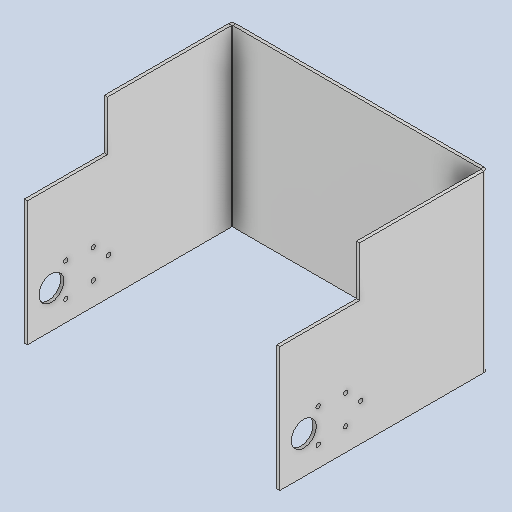
# Autodesk Inventor part: body_main_frame_new
Saved by Autodesk Inventor 2025.2 (Build 292293000, 293)
## iProperties
Created: 2025-05-30
Part Number: body_main_frame_new
Material: Aluminum 6061-AHC
Document SubType Name: Sheet Metal
Designer: chris
Density: 2.7 g/cm^3
Sheet Metal Rule: Default_mm
Appearance: Aluminum - Dark
Author: chris
Autodesk Inventor part; units mm, degrees
ref_plane "YZ Plane" through (0, 0, 0) normal (1, 0, 0) x (0, 1, 0)
ref_plane "XZ Plane" through (0, 0, 0) normal (0, 1, 0) x (-1, 0, 0)
ref_plane "XY Plane" through (0, 0, 0) normal (0, 0, 1) x (1, 0, 0)
sketch "Sketch4" plane through (0, 0, 0) normal (0, 0, 1) x (1, 0, 0)
  line L0 (-60, -42) -> (60, -42)
  line L1 (60, -42) -> (60, 42)
  line L2 (60, 42) -> (-60, 42)
  line L3 (-60, 42) -> (-60, -42)
  line L4 (-60, -42) -> (60, 42) construction
  line L5 (60, -42) -> (-60, 42) construction
  point P0 (0, 0)
  dimension "d13" = 120
  dimension "d14" = 84
  measures "d13" distance of L1.end L2.end
  measures "d14" distance of L0.end L1.end
extrude "Plate3" add sketch "Sketch4" along normal blind 1.5
sketch "Sketch5" plane through (61.5, 42, 0) normal (-1, 0, 0) x (0, -1, 0)
  line L0 (84, 0) -> (0, 0)
  line L1 (0, 0) -> (0, 100)
  line L2 (0, 100) -> (84, 100)
  line L3 (84, 100) -> (84, 0)
  line L4 (40, 5.9925) -> (78.4701, 5.9925)
  line L5 (78.4701, 5.9925) -> (78.4701, 78.464)
  line L6 (78.4701, 78.464) -> (40, 78.464)
  line L7 (40, 78.464) -> (40, 5.9925)
  constraints: 16 end point, 2 parallel, 1 horizontal, 1 perpendicular
edge flange "Flange2" height 100 angle 90 thickness 1.5 bend radius 0.31 thickness toward (-1, 0, 0) relief straight relief width 1.5 relief depth 0.75 corner gap 0.31 corner form 0 edges at (60, 0, 1.5) (-60, 0, 1.5) wall of the first edge with corners at (61.5, -42, 0) (61.5, 42, 0) (61.5, 42, 100) (61.5, -42, 100)
bend "Bend2"
corner "Corner2"
sketch "Sketch6" plane through (-61.5, -42, 100) normal (-1, 0, 0) x (0, 0, 1)
  line L0 (0, 60) -> (-38.5, 60)
  line L1 (-38.5, 60) -> (-38.5, 84)
  line L2 (-38.5, 84) -> (0, 84)
  line L3 (0, 84) -> (0, 60)
  line L4 (0, 84) -> (0, 0) projected
  line L5 (0, 0) -> (-98.19, 0) projected
  line L6 (-98.19, 84) -> (0, 84) projected
  point P0 (-100, 42)
  dimension "d26" = 38.5
  dimension "d27" = 24
  constraints: 8 end point, 2 collinear, 2 parallel, 1 horizontal, 1 perpendicular
  measures "d26" distance of L1.end L2.end
  measures "d27" distance of L2.end L0.start
extrude "Cut1" cut sketch "Sketch6" against normal blind 1.5
sketch "Sketch7" plane through (61.5, -42, 100) normal (1, 0, 0) x (0, 0, -1)
  line L0 (0, 60) -> (38.5, 60)
  line L1 (38.5, 60) -> (38.5, 84)
  line L2 (38.5, 84) -> (0, 84)
  line L3 (0, 84) -> (0, 60)
  line L4 (98.19, 0) -> (0, 0) projected
  line L5 (0, 0) -> (0, 84) projected
  line L6 (0, 84) -> (98.19, 84) projected
  point P0 (100, 42)
  dimension "d30" = 38.5
  dimension "d31" = 24
  constraints: 8 end point, 2 collinear, 2 parallel, 1 horizontal, 1 perpendicular
  measures "d30" distance of L1.end L2.end
  measures "d31" distance of L0.end L1.end
extrude "Cut2" cut sketch "Sketch7" against normal blind 1.5
sketch "Sketch8" plane through (-60, -42, 1.81) normal (1, 0, 0) x (0, 0, -1)
  point P0 (1.81, 42)
sketch "Sketch9" plane through (-60, -42, 1.81) normal (1, 0, 0) x (0, 0, -1)
  circle A0 centre (-79.79, 9.93) radius 0.7835 projected
  circle A1 centre (-66.57, 10.93) radius 0.7835 projected
  circle A2 centre (-59.27, 17.93) radius 0.7835 projected
  circle A3 centre (-79.79, 25.93) radius 0.7835 projected
  circle A4 centre (-66.57, 24.93) radius 0.7835 projected
  circle A5 centre (-86.69, 17.93) radius 6 projected
  point P0 (1.81, 42)
hole "Hole1" at (-60, -31.07, 68.38) at (-60, -24.07, 61.08) at (-60, -17.07, 68.38) at (-60, -16.07, 81.6) at (-60, -32.07, 81.6) direction (-1, 0, 0) diameter 2.1 depth 1.5
sketch "Sketch10" plane through (-60, -42, 1.81) normal (1, 0, 0) x (0, 0, -1)
  circle A0 centre (-86.69, 17.93) radius 6 projected
  point P0 (1.81, 42)
sketch "Sketch11" plane through (-60, -42, 1.81) normal (1, 0, 0) x (0, 0, -1)
  point P0 (1.81, 42)
extrude "Extrusion1" cut sketch "Sketch10" against normal blind 1.5
sketch "Sketch12" plane through (60, -42, 1.81) normal (-1, 0, 0) x (0, 0, 1)
  circle A0 centre (79.79, 25.93) radius 0.7835 projected
  circle A1 centre (79.79, 9.93) radius 0.7835 projected
  circle A2 centre (66.57, 10.93) radius 0.7835 projected
  circle A3 centre (59.27, 17.93) radius 0.7835 projected
  circle A4 centre (66.57, 24.93) radius 0.7835 projected
  point P0 (-1.81, 42)
hole "Hole2" at (60, -32.07, 81.6) at (60, -16.07, 81.6) at (60, -17.07, 68.38) at (60, -24.07, 61.08) at (60, -31.07, 68.38) direction (1, 0, 0) diameter 2.1 depth 1.5
sketch "Sketch13" plane through (60, -42, 1.81) normal (-1, 0, 0) x (0, 0, 1)
  circle A0 centre (86.69, 17.93) radius 6 projected
  point P0 (-1.81, 42)
extrude "Extrusion2" cut sketch "Sketch13" against normal blind 1.5
equation "\"d28\" = Thickness"
equation "\"d32\" = Thickness"
equation "\"d39\" = Thickness"
equation "\"d48\" = Thickness"
equation "\"d15\" = Thickness"
equation "\"d16\" = BendReliefWidth"
equation "\"d17\" = BendReliefDepth"
equation "\"d18\" = MinimumRemnant"
equation "\"d19\" = TransitionRadius"
equation "\"d22\" = BendRadius"
equation "\"d23\" = CornerReliefSize"
equation "\"d24\" = GapSize"
equation "\"d25\" = JacobiRadiusSize"
equation "\"BendReliefWidth\" = Thickness"
equation "\"BendReliefDepth\" = 0.5 * Thickness"
equation "\"CornerReliefSize\" = 4 * Thickness"
equation "\"MinimumRemnant\" = 2 * Thickness"
equation "\"TransitionRadius\" = BendRadius"
equation "\"JacobiRadiusSize\" = BendRadius"
equation "\"GapSize\" = Thickness"
equation "\"Thickness\" = 1.5"
equation "\"BendRadius\" = 0.31"
body "Solid2"
